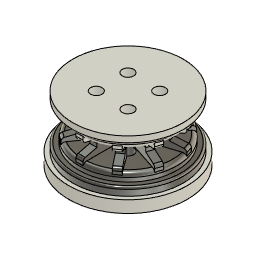
ball-chain-pulley (Autodesk Fusion 360 design; units mm, degrees)
Autodesk Fusion 360 part; units mm, degrees
sketch "Sketch1" plane through (0, 0, 0) normal (0, 0, 1) x (1, 0, 0) in component "Pulley"
ref_plane "WorkPlane1" through (0.9, 0, 0) normal (1, 0, 0) x (0, 1, 0) in component "Pulley"
sketch "Sketch2" plane through (0.9, 0, 0) normal (1, 0, 0) x (0, 1, 0) in component "Pulley"
  line L0 (12.2535, 0) -> (8.7535, 0)
  line L1 (8.7535, 0) -> (8.7535, 2.6)
  line L2 (8.7535, 2.6) -> (12.2535, 2.6)
  line L3 (12.2535, 0.214) -> (12.2535, 0)
  line L4 (8.7535, 1.6672) -> (11.6837, 0.942)
  arc A0 (12.2535, 0.214) -> (11.6837, 0.942) centre (11.5035, 0.214) ccw
  line L5 (8.7535, 0) -> (8.2535, 0)
  line L6 (8.2535, 0) -> (8.2535, 2.6)
  line L7 (8.2535, 2.6) -> (8.7535, 2.6)
  line L8 (8.7535, 2.6) -> (8.7535, 0)
  dimension "d4" = 3.5
  dimension "d5" = 2.6
  dimension "d6" = 8.7535
  dimension "d7" = 0.75
  constraint horizontal L0
  constraint vertical L1
  constraint horizontal L2
  constraint vertical L3
  constraint coincident L1 L4.start
  constraint coincident L2.end L3
  constraint tangent L4 A0
  constraint tangent L3 A0
  constraint horizontal L5
  constraint vertical L6
  constraint horizontal L7
  constraint vertical L8
  measures "d4" distance of L0.start L0.end
  measures "d5" distance of L0.start L2.end
  measures "d6" distance of origin L1
  measures "d7" radius of A0
extrude "Extrude1" add sketch "Sketch2" against normal blind 1.8 makes body 1 in component "Pulley"
extrude "Extrude2" add 1 faces at (0.3, 8.2535, 0.8667) along direction (0, -1, 0) blind 5 on bodies 1 bodies 1 in component "Pulley"
pattern_circular "C-Pattern1" count 10 over 360 about axis through (0, 0, 1.75) along (0, 0, 1) of bodies 1 makes body 2 at (-2.1639, 4.5095, 1.7333) makes body 3 at (-4.4013, 2.3764, 1.7333) makes body 4 at (-4.9575, -0.6645, 1.7333) makes body 5 at (-3.6201, -3.4515, 1.7333) makes body 6 at (-0.9, -4.9202, 1.7333) makes body 7 at (2.1639, -4.5095, 1.7333) makes body 8 at (4.4013, -2.3764, 1.7333) makes body 9 at (4.9575, 0.6645, 1.7333) makes body 10 at (3.6201, 3.4515, 1.7333) in component "Pulley"
sketch "Sketch3" plane through (0, 0, 0) normal (0, 0, 1) x (1, 0, 0) in component "Pulley"
  circle A0 centre (0, 0) radius 12.3535
  circle A1 centre (0, 0) radius 13.9235
  circle A2 centre (0, 0) radius 4.7535
  dimension "d16" = 24.707
  dimension "d17" = 1.57
  dimension "d18" = 9.507
  constraint coincident A0.centre A1.centre
  measures "d16" diameter of A0
  measures "d18" diameter of A2
extrude "Extrude3" add sketch "Sketch3" along normal blind 2.6 contours A2 bodies 1 6 8 9 10 7 2 3 4 5 in component "Pulley"
extrude "Extrude4" add sketch "Sketch3" against normal blind 3 contours A0 | A2 bodies 1 in component "Pulley"
extrude "Extrude5" add sketch "Sketch3" against normal blind 2 from surface at -2 contours A0 | A1 | A2 bodies 1 in component "Pulley"
fillet "Fillet1" radius 1 1 edges at (-11.5175, -4.4672, 0) on bodies 1 in component "Pulley"
fillet "Fillet2" radius 0.5 1 edges at (-12.9813, -5.035, -2) on bodies 1 in component "Pulley"
mirror "Mirror1" about plane through (0, 0, 2.6) normal (0, 0, 1) of bodies 1 makes body 11 in component "Pulley"
sketch "Sketch4" plane through (0, 0, 9.2) normal (0, 0, 1) x (-1, 0, 0) in component "Pulley"
  circle A0 centre (0, 0) radius 3
  line L0 (3, -2.598) -> (-3, -2.598)
  line L1 (-3, -2.598) -> (-3, 3)
  line L2 (-3, 3) -> (3, 3)
  line L3 (3, 3) -> (3, -2.598)
  circle A1 centre (0, 0) radius 4.7535 construction
  dimension "d33" = 6
  dimension "d34" = 6
  dimension "d35" = 5.598
  dimension "d36" = 3
  dimension "d39" = 9.507
  constraint coincident A0.centre A1.centre
  constraint horizontal L0
  constraint vertical L1
  constraint horizontal L2
  constraint vertical L3
  constraint tangent A0 L2
  constraint concentric A0 A1
  measures "d33" diameter of A0
  measures "d34" distance of L0.start L0.end
  measures "d35" distance of L0.start L2.end
  measures "d36" distance of A0.centre L3
  measures "d39" diameter of A1
sketch "Sketch1 (2)" plane through (0, 0, -4) normal (0, 0, -1) x (1, 0, 0) in component "Spacer"
  circle A0 centre (0, 0) radius 15
  dimension "d45" = 30
  constraint coincident A0.centre origin
  measures "d45" diameter of A0
extrude "Extrude1'" add sketch "Sketch1 (2)" along normal blind 17 separate body makes body 12 in component "Spacer"
extrude "Extrude6" cut sketch "Sketch4" against normal up to surface (28.7 mm away) from surface at -1.5 contours A0 L0 picked at (-0.1279, 0.5089) bodies 1 11 in component "Pulley"
extrude "Extrude2'" cut sketch "Sketch4" against normal up to surface (28.7 mm away) from surface at -1.5 contours A0 L0 picked at (-0.1279, 0.5089) bodies 12 in component "Spacer"
sketch "Sketch6" plane through (0, 0, 9.2) normal (0, 0, 1) x (-1, 0, 0) in component "Pulley"
  line L0 (-4, 4) -> (4, 4) construction
  line L1 (4, 4) -> (4, -4) construction
  line L2 (4, -4) -> (-4, -4) construction
  line L3 (-4, -4) -> (-4, 4) construction
  line L4 (-4, 4) -> (4, -4) construction
  line L5 (4, 4) -> (-4, -4) construction
  circle A0 centre (4, -4) radius 1.45
  circle A1 centre (4, -4) radius 1.45
  circle A2 centre (-4, -4) radius 1.45
  circle A3 centre (-4, -4) radius 1.45
  circle A4 centre (-4, 4) radius 1.45
  circle A5 centre (-4, 4) radius 1.45
  circle A6 centre (4, 4) radius 1.45
  circle A7 centre (4, 4) radius 1.45
  dimension "d54" = 8
  dimension "d55" = 8
  dimension "d56" = 2.9
  dimension "d57" = 2.9
  constraint horizontal L0
  constraint perpendicular L0 L1
  constraint parallel L0 L2
  constraint parallel L1 L3
  constraint coincident L4 origin
  constraint coincident L5 origin
  constraint coincident L1.end L2.start
  constraint concentric A0 A1
  constraint coincident L2.end L3.start
  constraint concentric A2 A3
  constraint coincident L0.start L3.end
  constraint concentric A4 A5
  constraint coincident L0.end L1.start
  constraint concentric A6 A7
  constraint equal A0 A2
  constraint equal A0 A4
  constraint equal A0 A6
  constraint equal A1 A7
  constraint equal A1 A5
  constraint equal A1 A3
  measures "d54" distance of L1.end L2.end
  measures "d55" distance of L0.end L1.end
  measures "d56" diameter of A0
  measures "d57" diameter of A1
extrude "Extrude7" cut sketch "Sketch6" against normal blind 13.2 bodies 1 11 in component "Pulley"
extrude "Extrude8" [suppressed] in component "Pulley"
extrude "Extrude3'" cut sketch "Sketch6" against normal up to surface (30.2 mm away) bodies 12 in component "Spacer"
move_face "OffsetFaces1" offset -0.09 4 faces at (2.9851, 0.2986, 4.3) (-0.5, 2.598, 6) (2.9851, 0.2986, -1.8) (0.5, 2.598, -1.8) on bodies 1 11 in component "Pulley"
move_face "OffsetFaces1'" offset -0.09 2 faces at (2.9963, 0.1494, -15.3333) (-0.5, 2.598, -9.6667) on bodies 12 in component "Spacer"
extrude "Extrude4'" cut 1 faces at (-8.4654, 0, -21) along direction (0, 0, 1) blind 14 on bodies 12 bodies 12 in component "Spacer"
copy_body "Body->Comp1" bodies 11 removing the originals makes body 13 in component "TopHalf"
copy_body "Body->Comp2" bodies 1 removing the originals makes body 14 in component "BottomHalf"
component "Pulley" placed x (1, 0, 0) y (0, 1, 0) z (0, 0, 1) at (0, 0, 0)
component "Spacer" placed x (1, 0, 0) y (0, 1, 0) z (0, 0, 1) at (0, 0, 0)
component "TopHalf" placed x (1, 0, 0) y (0, 1, 0) z (0, 0, 1) at (0, 0, 0) in component "Pulley"
component "BottomHalf" placed x (1, 0, 0) y (0, 1, 0) z (0, 0, 1) at (0, 0, 0) in component "Pulley"
equation "齿间距 = 5.5 mm"
equation "d3 = ( 1.8 / 2 ) * 1 mm"
equation "d5 = ( 5.2 / 2 ) * 1 mm"
equation "d6 = ( ( 齿间距 * 齿数 ) / PI ) / 2"
equation "齿数 = 10"
equation "d14 = 齿数"
equation "d16 = ( ( 齿间距 * 齿数 ) / PI ) + 7.2 mm"
equation "d18 = ( ( 齿间距 * 齿数 ) / PI ) - 8 mm"
equation "d33 = 电机D轴直径"
equation "d34 = 电机D轴直径"
equation "d35 = 电机D轴平面同圆周距离"
equation "d36 = 电机D轴直径 / 2"
equation "电机D轴直径 = 6 mm"
equation "电机D轴平面同圆周距离 = 5.598 mm"
equation "d39 = ( ( 齿间距 * 齿数 ) / PI ) - 8 mm"
equation "d56 = 紧固螺丝小孔直径"
equation "d57 = 紧固螺丝大孔直径"
equation "紧固螺丝小孔直径 = 2.9 mm"
equation "紧固螺丝大孔直径 = 2.9 mm"
equation "紧固螺丝大孔深度 = 13.2 mm"
equation "d67 = -紧固螺丝大孔深度"
